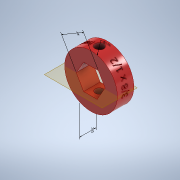
# Autodesk Inventor part: 3_8x1_2-hexBearingSplitA
Saved by Autodesk Inventor 2022.1 (Build 261234000, 234)
## iProperties
Created: 2020-11-08
Part Number: 3_8x1_2-hexBearingSplitA
Material: PC/ABS Plastic
Document SubType Name: Modeling
Designer: robst
Density: 0.357273 g/cm^3
Appearance: Red
Author: robst
Autodesk Inventor part; units mm, degrees
ref_plane "YZ Plane" through (0, 0, 0) normal (1, 0, 0) x (0, 1, 0)
ref_plane "XY Plane" through (0, 0, 0) normal (0, 0, 1) x (1, 0, 0)
sketch "Sketch1" plane through (0, 0, 0) normal (0, 0, 1) x (1, 0, 0)
  line L0 (3.6662, 6.35) -> (7.3323, 0)
  line L1 (7.3323, 0) -> (3.6662, -6.35)
  line L2 (3.6662, -6.35) -> (-3.6662, -6.35)
  line L3 (-3.6662, -6.35) -> (-7.3323, 0)
  line L4 (-7.3323, 0) -> (-3.6662, 6.35)
  line L5 (-3.6662, 6.35) -> (3.6662, 6.35)
  circle A0 centre (0, 0) radius 14.2875
  circle A1 centre (0, 0) radius 7.3323 construction
  dimension "d0" = 12.7
  dimension "d2" = 28.575
  dimension "d3" = 6.9551
  constraints: 12 end point, 3 coincident, 1 centre point, 1 horizontal, 1 horizontal alignment, 15 other
  measures "d0" distance between parallel lines of L2 L5
  measures "d2" diameter of A0
extrude "Extrusion1" add sketch "Sketch1" against normal blind 9.525
thicken "Thicken2" operation add thickness 0.5715 both sides no extend neighbours yes toward (-0.8660254, -0.5, 0) faces at (-4.8882, -4.2333, -3.175) (-6.1103, 2.1167, -3.175) (-1.2221, 6.35, -3.175) (4.8882, 4.2333, -3.175) (7.8832, 4.3299, 0) (1.2221, -6.35, -3.175)
ref_plane "Work Plane1" through (0, 14.2875, 0) normal (0, 1, 0) x (-1, 0, 0)
sketch "Sketch2" plane through (0, 14.2875, 0) normal (0, 1, 0) x (-1, 0, 0)
  line L0 (0, -6.9215) -> (-25.4, -6.9215) construction
  line L1 (14.2875, -0.5715) -> (-14.2875, -0.5715) construction
  spline S0 degree 2 poles (-24.3116, -3.4125) (-24.4274, -3.4125) (-24.6564, -3.4691) (-24.7671, -3.5129) knots 0 0 0 1 2 2 2
  spline S1 degree 2 poles (-24.7671, -3.5129) (-24.87, -3.5566) (-25.0218, -3.6492) (-25.081, -3.6904) knots 0 0 0 1 2 2 2
  line L2 (-25.081, -3.6904) -> (-25.1067, -3.6904)
  line L3 (-25.1067, -3.6904) -> (-25.1067, -3.2401)
  spline S2 degree 2 poles (-25.1067, -3.2401) (-24.9677, -3.1655) (-24.4918, -3.0446) (-24.2782, -3.0446) knots 0 0 0 1 2 2 2
  spline S3 degree 2 poles (-24.2782, -3.0446) (-24.0621, -3.0446) (-23.7405, -3.1321) (-23.6092, -3.2247) knots 0 0 0 1 2 2 2
  spline S4 degree 2 poles (-23.6092, -3.2247) (-23.4703, -3.3251) (-23.3262, -3.6158) (-23.3262, -3.8113) knots 0 0 0 1 2 2 2
  spline S5 degree 2 poles (-23.3262, -3.8113) (-23.3262, -4.0738) (-23.671, -4.47) (-23.9128, -4.5215) knots 0 0 0 1 2 2 2
  line L4 (-23.9128, -4.5215) -> (-23.9128, -4.5523)
  spline S6 degree 2 poles (-23.9128, -4.5523) (-23.8125, -4.5729) (-23.5835, -4.6656) (-23.4857, -4.7582) knots 0 0 0 1 2 2 2
  spline S7 degree 2 poles (-23.4857, -4.7582) (-23.388, -4.8482) (-23.2645, -5.1364) (-23.2645, -5.3448) knots 0 0 0 1 2 2 2
  spline S8 degree 2 poles (-23.2645, -5.3448) (-23.2645, -5.5584) (-23.4111, -5.9211) (-23.5449, -6.0601) knots 0 0 0 1 2 2 2
  spline S9 degree 2 poles (-23.5449, -6.0601) (-23.6839, -6.2042) (-24.0775, -6.3534) (-24.3271, -6.3534) knots 0 0 0 1 2 2 2
  spline S10 degree 2 poles (-24.3271, -6.3534) (-24.5664, -6.3534) (-25.0346, -6.2376) (-25.1942, -6.1579) knots 0 0 0 1 2 2 2
  line L5 (-25.1942, -6.1579) -> (-25.1942, -5.7076)
  line L6 (-25.1942, -5.7076) -> (-25.1633, -5.7076)
  spline S11 degree 2 poles (-25.1633, -5.7076) (-25.0295, -5.8054) (-24.5767, -5.9855) (-24.3528, -5.9855) knots 0 0 0 1 2 2 2
  spline S12 degree 2 poles (-24.3528, -5.9855) (-24.2216, -5.9855) (-23.9592, -5.9031) (-23.8717, -5.8079) knots 0 0 0 1 2 2 2
  spline S13 degree 2 poles (-23.8717, -5.8079) (-23.7868, -5.7127) (-23.6967, -5.4863) (-23.6967, -5.3139) knots 0 0 0 1 2 2 2
  spline S14 degree 2 poles (-23.6967, -5.3139) (-23.6967, -5.1415) (-23.7971, -4.9177) (-23.8871, -4.8534) knots 0 0 0 1 2 2 2
  spline S15 degree 2 poles (-23.8871, -4.8534) (-23.9772, -4.7891) (-24.2216, -4.7402) (-24.3657, -4.7402) knots 0 0 0 1 2 2 2
  line L7 (-24.3657, -4.7402) -> (-24.5458, -4.7402)
  line L8 (-24.5458, -4.7402) -> (-24.5458, -4.3877)
  line L9 (-24.5458, -4.3877) -> (-24.4043, -4.3877)
  spline S16 degree 2 poles (-24.4043, -4.3877) (-24.1187, -4.3877) (-23.7585, -4.1149) (-23.7585, -3.8551) knots 0 0 0 1 2 2 2
  spline S17 degree 2 poles (-23.7585, -3.8551) (-23.7585, -3.7341) (-23.8511, -3.5618) (-23.9257, -3.5103) knots 0 0 0 1 2 2 2
  spline S18 degree 2 poles (-23.9257, -3.5103) (-24.0055, -3.4563) (-24.201, -3.4125) (-24.3116, -3.4125) knots 0 0 0 1 2 2 2
  line L10 (-21.466, -2.97) -> (-22.7087, -6.976)
  line L11 (-22.7087, -6.976) -> (-23.0689, -6.976)
  line L12 (-23.0689, -6.976) -> (-21.8313, -2.97)
  line L13 (-21.8313, -2.97) -> (-21.466, -2.97)
  spline S19 degree 2 poles (-20.1564, -6.3585) (-20.3931, -6.3585) (-20.7816, -6.217) (-20.9179, -6.0858) knots 0 0 0 1 2 2 2
  spline S20 degree 2 poles (-20.9179, -6.0858) (-21.0517, -5.9572) (-21.1907, -5.6072) (-21.1907, -5.4091) knots 0 0 0 1 2 2 2
  spline S21 degree 2 poles (-21.1907, -5.4091) (-21.1907, -5.1518) (-20.9154, -4.7196) (-20.6529, -4.5909) knots 0 0 0 1 2 2 2
  line L14 (-20.6529, -4.5909) -> (-20.6529, -4.5781)
  spline S22 degree 2 poles (-20.6529, -4.5781) (-20.8871, -4.4417) (-21.1135, -4.1175) (-21.1135, -3.8757) knots 0 0 0 1 2 2 2
  spline S23 degree 2 poles (-21.1135, -3.8757) (-21.1135, -3.518) (-20.5732, -3.0395) (-20.1564, -3.0395) knots 0 0 0 1 2 2 2
  spline S24 degree 2 poles (-20.1564, -3.0395) (-19.7241, -3.0395) (-19.2018, -3.4923) (-19.2018, -3.8474) knots 0 0 0 1 2 2 2
  spline S25 degree 2 poles (-19.2018, -3.8474) (-19.2018, -4.0609) (-19.4514, -4.4777) (-19.6855, -4.5961) knots 0 0 0 1 2 2 2
  line L15 (-19.6855, -4.5961) -> (-19.6855, -4.6089)
  spline S26 degree 2 poles (-19.6855, -4.6089) (-19.4076, -4.7376) (-19.122, -5.1081) (-19.122, -5.4014) knots 0 0 0 1 2 2 2
  spline S27 degree 2 poles (-19.122, -5.4014) (-19.122, -5.8079) (-19.7138, -6.3585) (-20.1564, -6.3585) knots 0 0 0 1 2 2 2
  spline S28 degree 2 poles (-19.5594, -5.4426) (-19.5594, -5.247) (-19.7138, -5.0155) (-19.9325, -4.8971) knots 0 0 0 1 2 2 2
  spline S29 degree 2 poles (-19.9325, -4.8971) (-20.0046, -4.8559) (-20.2464, -4.7608) (-20.3982, -4.699) knots 0 0 0 1 2 2 2
  spline S30 degree 2 poles (-20.3982, -4.699) (-20.5732, -4.8148) (-20.761, -5.1596) (-20.761, -5.3783) knots 0 0 0 1 2 2 2
  spline S31 degree 2 poles (-20.761, -5.3783) (-20.761, -5.6664) (-20.4137, -6.0421) (-20.1512, -6.0421) knots 0 0 0 1 2 2 2
  spline S32 degree 2 poles (-20.1512, -6.0421) (-19.8836, -6.0421) (-19.5594, -5.7205) (-19.5594, -5.4426) knots 0 0 0 1 2 2 2
  spline S33 degree 2 poles (-19.6186, -3.8525) (-19.6186, -3.639) (-19.9042, -3.3534) (-20.1589, -3.3534) knots 0 0 0 1 2 2 2
  spline S34 degree 2 poles (-20.1589, -3.3534) (-20.3905, -3.3534) (-20.6864, -3.6081) (-20.6864, -3.8268) knots 0 0 0 1 2 2 2
  spline S35 degree 2 poles (-20.6864, -3.8268) (-20.6864, -3.9837) (-20.5346, -4.2024) (-20.3828, -4.2899) knots 0 0 0 1 2 2 2
  spline S36 degree 2 poles (-20.3828, -4.2899) (-20.3185, -4.3259) (-20.0457, -4.452) (-19.9351, -4.488) knots 0 0 0 1 2 2 2
  spline S37 degree 2 poles (-19.9351, -4.488) (-19.7498, -4.3465) (-19.6186, -4.0455) (-19.6186, -3.8525) knots 0 0 0 1 2 2 2
  line L16 (-15.4608, -6.2865) -> (-15.9522, -6.2865)
  line L17 (-15.9522, -6.2865) -> (-16.5311, -5.3911)
  line L18 (-16.5311, -5.3911) -> (-17.1254, -6.2865)
  line L19 (-17.1254, -6.2865) -> (-17.5809, -6.2865)
  line L20 (-17.5809, -6.2865) -> (-16.7549, -5.1055)
  line L21 (-16.7549, -5.1055) -> (-17.5731, -3.904)
  line L22 (-17.5731, -3.904) -> (-17.0817, -3.904)
  line L23 (-17.0817, -3.904) -> (-16.5054, -4.7916)
  line L24 (-16.5054, -4.7916) -> (-15.9162, -3.904)
  line L25 (-15.9162, -3.904) -> (-15.4608, -3.904)
  line L26 (-15.4608, -3.904) -> (-16.2815, -5.0798)
  line L27 (-16.2815, -5.0798) -> (-15.4608, -6.2865)
  line L28 (-12.0465, -6.2865) -> (-13.5954, -6.2865)
  line L29 (-13.5954, -6.2865) -> (-13.5954, -5.9623)
  line L30 (-13.5954, -5.9623) -> (-13.019, -5.9623)
  line L31 (-13.019, -5.9623) -> (-13.019, -3.8345)
  line L32 (-13.019, -3.8345) -> (-13.5954, -3.8345)
  line L33 (-13.5954, -3.8345) -> (-13.5954, -3.5438)
  spline S38 degree 2 poles (-13.5954, -3.5438) (-13.2686, -3.5438) (-12.9599, -3.3585) (-12.9393, -3.1012) knots 0 0 0 1 2 2 2
  line L34 (-12.9393, -3.1012) -> (-12.6099, -3.1012)
  line L35 (-12.6099, -3.1012) -> (-12.6099, -5.9623)
  line L36 (-12.6099, -5.9623) -> (-12.0465, -5.9623)
  line L37 (-12.0465, -5.9623) -> (-12.0465, -6.2865)
  line L38 (-10.1425, -2.97) -> (-11.3852, -6.976)
  line L39 (-11.3852, -6.976) -> (-11.7454, -6.976)
  line L40 (-11.7454, -6.976) -> (-10.5079, -2.97)
  line L41 (-10.5079, -2.97) -> (-10.1425, -2.97)
  line L42 (-7.8346, -6.2865) -> (-9.7926, -6.2865)
  line L43 (-9.7926, -6.2865) -> (-9.7926, -5.8362)
  spline S39 degree 2 poles (-9.7926, -5.8362) (-9.5816, -5.6381) (-9.206, -5.2702) (-9.0259, -5.0721) knots 0 0 0 1 2 2 2
  spline S40 degree 2 poles (-9.0259, -5.0721) (-8.6631, -4.6733) (-8.3981, -4.1947) (-8.3981, -3.94) knots 0 0 0 1 2 2 2
  spline S41 degree 2 poles (-8.3981, -3.94) (-8.3981, -3.8062) (-8.4804, -3.6055) (-8.555, -3.5412) knots 0 0 0 1 2 2 2
  spline S42 degree 2 poles (-8.555, -3.5412) (-8.6296, -3.4769) (-8.8252, -3.4125) (-8.9435, -3.4125) knots 0 0 0 1 2 2 2
  spline S43 degree 2 poles (-8.9435, -3.4125) (-9.0567, -3.4125) (-9.2883, -3.4691) (-9.3938, -3.5129) knots 0 0 0 1 2 2 2
  spline S44 degree 2 poles (-9.3938, -3.5129) (-9.4838, -3.5489) (-9.6511, -3.6518) (-9.7025, -3.6878) knots 0 0 0 1 2 2 2
  line L44 (-9.7025, -3.6878) -> (-9.7257, -3.6878)
  line L45 (-9.7257, -3.6878) -> (-9.7257, -3.235)
  spline S45 degree 2 poles (-9.7257, -3.235) (-9.5945, -3.1707) (-9.1236, -3.0446) (-8.9126, -3.0446) knots 0 0 0 1 2 2 2
  spline S46 degree 2 poles (-8.9126, -3.0446) (-8.4675, -3.0446) (-7.9658, -3.5155) (-7.9658, -3.9168) knots 0 0 0 1 2 2 2
  spline S47 degree 2 poles (-7.9658, -3.9168) (-7.9658, -4.1047) (-8.0533, -4.4186) (-8.1305, -4.5523) knots 0 0 0 1 2 2 2
  spline S48 degree 2 poles (-8.1305, -4.5523) (-8.2077, -4.6913) (-8.4315, -4.964) (-8.555, -5.0952) knots 0 0 0 1 2 2 2
  spline S49 degree 2 poles (-8.555, -5.0952) (-8.7557, -5.3139) (-9.2471, -5.7822) (-9.3938, -5.9186) knots 0 0 0 1 2 2 2
  line L46 (-9.3938, -5.9186) -> (-7.8346, -5.9186)
  line L47 (-7.8346, -5.9186) -> (-7.8346, -6.2865)
  line L48 (5.4289, -6.2865) -> (5.0275, -6.2865)
  line L49 (5.0275, -6.2865) -> (5.0275, -4.928)
  spline S50 degree 2 poles (5.0275, -4.928) (5.0275, -4.7633) (4.9966, -4.4803) (4.9503, -4.3954) knots 0 0 0 1 2 2 2
  spline S51 degree 2 poles (4.9503, -4.3954) (4.9014, -4.3053) (4.7265, -4.2179) (4.5772, -4.2179) knots 0 0 0 1 2 2 2
  spline S52 degree 2 poles (4.5772, -4.2179) (4.428, -4.2179) (4.1115, -4.3774) (3.9597, -4.506) knots 0 0 0 1 2 2 2
  line L50 (3.9597, -4.506) -> (3.9597, -6.2865)
  line L51 (3.9597, -6.2865) -> (3.5584, -6.2865)
  line L52 (3.5584, -6.2865) -> (3.5584, -2.97)
  line L53 (3.5584, -2.97) -> (3.9597, -2.97)
  line L54 (3.9597, -2.97) -> (3.9597, -4.169)
  spline S53 degree 2 poles (3.9597, -4.169) (4.1398, -4.0069) (4.4872, -3.8371) (4.6827, -3.8371) knots 0 0 0 1 2 2 2
  spline S54 degree 2 poles (4.6827, -3.8371) (5.0327, -3.8371) (5.4289, -4.3002) (5.4289, -4.7402) knots 0 0 0 1 2 2 2
  line L55 (5.4289, -4.7402) -> (5.4289, -6.2865)
  spline S55 degree 2 poles (7.0267, -6.3405) (6.4555, -6.3405) (5.8277, -5.6999) (5.8277, -5.1081) knots 0 0 0 1 2 2 2
  spline S56 degree 2 poles (5.8277, -5.1081) (5.8277, -4.5266) (6.4375, -3.8371) (6.9289, -3.8371) knots 0 0 0 1 2 2 2
  spline S57 degree 2 poles (6.9289, -3.8371) (7.1502, -3.8371) (7.4924, -3.9657) (7.6185, -4.1021) knots 0 0 0 1 2 2 2
  spline S58 degree 2 poles (7.6185, -4.1021) (7.7471, -4.2384) (7.8835, -4.6321) (7.8835, -4.9177) knots 0 0 0 1 2 2 2
  line L56 (7.8835, -4.9177) -> (7.8835, -5.1364)
  line L57 (7.8835, -5.1364) -> (6.2342, -5.1364)
  spline S59 degree 2 poles (6.2342, -5.1364) (6.2342, -5.5506) (6.651, -5.9906) (7.0215, -5.9906) knots 0 0 0 1 2 2 2
  spline S60 degree 2 poles (7.0215, -5.9906) (7.1528, -5.9906) (7.4075, -5.9314) (7.5104, -5.8851) knots 0 0 0 1 2 2 2
  spline S61 degree 2 poles (7.5104, -5.8851) (7.6185, -5.8337) (7.7677, -5.7436) (7.8166, -5.7024) knots 0 0 0 1 2 2 2
  line L58 (7.8166, -5.7024) -> (7.8397, -5.7024)
  line L59 (7.8397, -5.7024) -> (7.8397, -6.1398)
  spline S62 degree 2 poles (7.8397, -6.1398) (7.7703, -6.1681) (7.5593, -6.2505) (7.4769, -6.2736) knots 0 0 0 1 2 2 2
  spline S63 degree 2 poles (7.4769, -6.2736) (7.3612, -6.3071) (7.1708, -6.3405) (7.0267, -6.3405) knots 0 0 0 1 2 2 2
  spline S64 degree 2 poles (7.4924, -4.8302) (7.4872, -4.6681) (7.4203, -4.4314) (7.356, -4.3517) knots 0 0 0 1 2 2 2
  spline S65 degree 2 poles (7.356, -4.3517) (7.2865, -4.2616) (7.0678, -4.1664) (6.9058, -4.1664) knots 0 0 0 1 2 2 2
  spline S66 degree 2 poles (6.9058, -4.1664) (6.7462, -4.1664) (6.5224, -4.2616) (6.4298, -4.3542) knots 0 0 0 1 2 2 2
  spline S67 degree 2 poles (6.4298, -4.3542) (6.3397, -4.4494) (6.2471, -4.6784) (6.2342, -4.8302) knots 0 0 0 1 2 2 2
  line L60 (6.2342, -4.8302) -> (7.4924, -4.8302)
  line L61 (10.1399, -6.2865) -> (9.6485, -6.2865)
  line L62 (9.6485, -6.2865) -> (9.0696, -5.3911)
  line L63 (9.0696, -5.3911) -> (8.4752, -6.2865)
  line L64 (8.4752, -6.2865) -> (8.0198, -6.2865)
  line L65 (8.0198, -6.2865) -> (8.8457, -5.1055)
  line L66 (8.8457, -5.1055) -> (8.0276, -3.904)
  line L67 (8.0276, -3.904) -> (8.519, -3.904)
  line L68 (8.519, -3.904) -> (9.0953, -4.7916)
  line L69 (9.0953, -4.7916) -> (9.6845, -3.904)
  line L70 (9.6845, -3.904) -> (10.1399, -3.904)
  line L71 (10.1399, -3.904) -> (9.3192, -5.0798)
  line L72 (9.3192, -5.0798) -> (10.1399, -6.2865)
  spline S68 degree 2 poles (13.8115, -5.0566) (13.8115, -5.6407) (13.2455, -6.3534) (12.8184, -6.3534) knots 0 0 0 1 2 2 2
  spline S69 degree 2 poles (12.8184, -6.3534) (12.6254, -6.3534) (12.3501, -6.2582) (12.2163, -6.1759) knots 0 0 0 1 2 2 2
  line L73 (12.2163, -6.1759) -> (12.1906, -6.2865)
  line L74 (12.1906, -6.2865) -> (11.8149, -6.2865)
  line L75 (11.8149, -6.2865) -> (11.8149, -2.97)
  line L76 (11.8149, -2.97) -> (12.2163, -2.97)
  line L77 (12.2163, -2.97) -> (12.2163, -4.1535)
  spline S70 degree 2 poles (12.2163, -4.1535) (12.3681, -4.0172) (12.7206, -3.8371) (12.9444, -3.8371) knots 0 0 0 1 2 2 2
  spline S71 degree 2 poles (12.9444, -3.8371) (13.3484, -3.8371) (13.8115, -4.4829) (13.8115, -5.0566) knots 0 0 0 1 2 2 2
  spline S72 degree 2 poles (13.3973, -5.0875) (13.3973, -4.6604) (13.1374, -4.2179) (12.8492, -4.2179) knots 0 0 0 1 2 2 2
  spline S73 degree 2 poles (12.8492, -4.2179) (12.6871, -4.2179) (12.3527, -4.3722) (12.2163, -4.4906) knots 0 0 0 1 2 2 2
  line L78 (12.2163, -4.4906) -> (12.2163, -5.8568)
  spline S74 degree 2 poles (12.2163, -5.8568) (12.3681, -5.9314) (12.6022, -5.9932) (12.7412, -5.9932) knots 0 0 0 1 2 2 2
  spline S75 degree 2 poles (12.7412, -5.9932) (13.0473, -5.9932) (13.3973, -5.5584) (13.3973, -5.0875) knots 0 0 0 1 2 2 2
  line L79 (16.0808, -6.2865) -> (15.6795, -6.2865)
  line L80 (15.6795, -6.2865) -> (15.6795, -6.0241)
  spline S76 degree 2 poles (15.6795, -6.0241) (15.4942, -6.1862) (15.1623, -6.3534) (14.9565, -6.3534) knots 0 0 0 1 2 2 2
  spline S77 degree 2 poles (14.9565, -6.3534) (14.8021, -6.3534) (14.5268, -6.2505) (14.4264, -6.1398) knots 0 0 0 1 2 2 2
  spline S78 degree 2 poles (14.4264, -6.1398) (14.3235, -6.0292) (14.2103, -5.6922) (14.2103, -5.4503) knots 0 0 0 1 2 2 2
  line L81 (14.2103, -5.4503) -> (14.2103, -3.904)
  line L82 (14.2103, -3.904) -> (14.6117, -3.904)
  line L83 (14.6117, -3.904) -> (14.6117, -5.2625)
  spline S79 degree 2 poles (14.6117, -5.2625) (14.6117, -5.4529) (14.64, -5.7024) (14.6889, -5.7951) knots 0 0 0 1 2 2 2
  spline S80 degree 2 poles (14.6889, -5.7951) (14.7378, -5.8877) (14.905, -5.9726) (15.062, -5.9726) knots 0 0 0 1 2 2 2
  spline S81 degree 2 poles (15.062, -5.9726) (15.2086, -5.9726) (15.5405, -5.8054) (15.6795, -5.6844) knots 0 0 0 1 2 2 2
  line L84 (15.6795, -5.6844) -> (15.6795, -3.904)
  line L85 (15.6795, -3.904) -> (16.0808, -3.904)
  line L86 (16.0808, -3.904) -> (16.0808, -6.2865)
  spline S82 degree 2 poles (17.3055, -6.3431) (17.0663, -6.3431) (16.652, -6.2145) (16.5157, -6.1424) knots 0 0 0 1 2 2 2
  line L87 (16.5157, -6.1424) -> (16.5157, -5.6922)
  line L88 (16.5157, -5.6922) -> (16.5362, -5.6922)
  spline S83 degree 2 poles (16.5362, -5.6922) (16.5877, -5.7333) (16.7266, -5.8311) (16.8424, -5.8851) knots 0 0 0 1 2 2 2
  spline S84 degree 2 poles (16.8424, -5.8851) (16.9428, -5.934) (17.1898, -6.0061) (17.321, -6.0061) knots 0 0 0 1 2 2 2
  spline S85 degree 2 poles (17.321, -6.0061) (17.4162, -6.0061) (17.6349, -5.9623) (17.6863, -5.9263) knots 0 0 0 1 2 2 2
  spline S86 degree 2 poles (17.6863, -5.9263) (17.761, -5.8774) (17.8279, -5.7668) (17.8279, -5.6536) knots 0 0 0 1 2 2 2
  spline S87 degree 2 poles (17.8279, -5.6536) (17.8279, -5.512) (17.6735, -5.3654) (17.4754, -5.3165) knots 0 0 0 1 2 2 2
  spline S88 degree 2 poles (17.4754, -5.3165) (17.3982, -5.2985) (17.1512, -5.247) (17.0457, -5.2187) knots 0 0 0 1 2 2 2
  spline S89 degree 2 poles (17.0457, -5.2187) (16.773, -5.139) (16.526, -4.8096) (16.526, -4.5755) knots 0 0 0 1 2 2 2
  spline S90 degree 2 poles (16.526, -4.5755) (16.526, -4.2513) (17.0122, -3.8474) (17.4136, -3.8474) knots 0 0 0 1 2 2 2
  spline S91 degree 2 poles (17.4136, -3.8474) (17.6117, -3.8474) (18.0131, -3.9451) (18.1495, -4.0197) knots 0 0 0 1 2 2 2
  line L89 (18.1495, -4.0197) -> (18.1495, -4.4494)
  line L90 (18.1495, -4.4494) -> (18.1289, -4.4494)
  spline S92 degree 2 poles (18.1289, -4.4494) (17.9745, -4.3259) (17.5989, -4.1844) (17.4059, -4.1844) knots 0 0 0 1 2 2 2
  spline S93 degree 2 poles (17.4059, -4.1844) (17.2078, -4.1844) (16.935, -4.3517) (16.935, -4.5189) knots 0 0 0 1 2 2 2
  spline S94 degree 2 poles (16.935, -4.5189) (16.935, -4.6707) (17.0971, -4.8174) (17.2772, -4.8637) knots 0 0 0 1 2 2 2
  spline S95 degree 2 poles (17.2772, -4.8637) (17.3647, -4.8868) (17.586, -4.9331) (17.7069, -4.9614) knots 0 0 0 1 2 2 2
  spline S96 degree 2 poles (17.7069, -4.9614) (17.9694, -5.0283) (18.237, -5.3345) (18.237, -5.5995) knots 0 0 0 1 2 2 2
  spline S97 degree 2 poles (18.237, -5.5995) (18.237, -5.7539) (18.116, -6.0266) (17.9977, -6.127) knots 0 0 0 1 2 2 2
  spline S98 degree 2 poles (17.9977, -6.127) (17.8716, -6.2325) (17.55, -6.3431) (17.3055, -6.3431) knots 0 0 0 1 2 2 2
  line L91 (20.4805, -6.2865) -> (20.0792, -6.2865)
  line L92 (20.0792, -6.2865) -> (20.0792, -4.928)
  spline S99 degree 2 poles (20.0792, -4.928) (20.0792, -4.7633) (20.0483, -4.4803) (20.002, -4.3954) knots 0 0 0 1 2 2 2
  spline S100 degree 2 poles (20.002, -4.3954) (19.9531, -4.3053) (19.7781, -4.2179) (19.6289, -4.2179) knots 0 0 0 1 2 2 2
  spline S101 degree 2 poles (19.6289, -4.2179) (19.4797, -4.2179) (19.1632, -4.3774) (19.0114, -4.506) knots 0 0 0 1 2 2 2
  line L93 (19.0114, -4.506) -> (19.0114, -6.2865)
  line L94 (19.0114, -6.2865) -> (18.61, -6.2865)
  line L95 (18.61, -6.2865) -> (18.61, -2.97)
  line L96 (18.61, -2.97) -> (19.0114, -2.97)
  line L97 (19.0114, -2.97) -> (19.0114, -4.169)
  spline S102 degree 2 poles (19.0114, -4.169) (19.1915, -4.0069) (19.5389, -3.8371) (19.7344, -3.8371) knots 0 0 0 1 2 2 2
  spline S103 degree 2 poles (19.7344, -3.8371) (20.0843, -3.8371) (20.4805, -4.3002) (20.4805, -4.7402) knots 0 0 0 1 2 2 2
  line L98 (20.4805, -4.7402) -> (20.4805, -6.2865)
  line L99 (21.4531, -6.2865) -> (21.0517, -6.2865)
  line L100 (21.0517, -6.2865) -> (21.0517, -3.904)
  line L101 (21.0517, -3.904) -> (21.4531, -3.904)
  line L102 (21.4531, -3.904) -> (21.4531, -6.2865)
  line L103 (21.4814, -3.5077) -> (21.026, -3.5077)
  line L104 (21.026, -3.5077) -> (21.026, -3.0909)
  line L105 (21.026, -3.0909) -> (21.4814, -3.0909)
  line L106 (21.4814, -3.0909) -> (21.4814, -3.5077)
  line L107 (23.9128, -6.2865) -> (23.5115, -6.2865)
  line L108 (23.5115, -6.2865) -> (23.5115, -4.928)
  spline S104 degree 2 poles (23.5115, -4.928) (23.5115, -4.7633) (23.4806, -4.4803) (23.4343, -4.3954) knots 0 0 0 1 2 2 2
  spline S105 degree 2 poles (23.4343, -4.3954) (23.3854, -4.3053) (23.2104, -4.2179) (23.0612, -4.2179) knots 0 0 0 1 2 2 2
  spline S106 degree 2 poles (23.0612, -4.2179) (22.912, -4.2179) (22.5955, -4.3774) (22.4437, -4.506) knots 0 0 0 1 2 2 2
  line L109 (22.4437, -4.506) -> (22.4437, -6.2865)
  line L110 (22.4437, -6.2865) -> (22.0423, -6.2865)
  line L111 (22.0423, -6.2865) -> (22.0423, -3.904)
  line L112 (22.0423, -3.904) -> (22.4437, -3.904)
  line L113 (22.4437, -3.904) -> (22.4437, -4.169)
  spline S107 degree 2 poles (22.4437, -4.169) (22.6238, -4.0069) (22.9711, -3.8371) (23.1667, -3.8371) knots 0 0 0 1 2 2 2
  spline S108 degree 2 poles (23.1667, -3.8371) (23.5166, -3.8371) (23.9128, -4.3002) (23.9128, -4.7402) knots 0 0 0 1 2 2 2
  line L114 (23.9128, -4.7402) -> (23.9128, -6.2865)
  spline S109 degree 2 poles (24.5612, -6.6673) (24.6024, -6.6853) (24.7593, -6.7419) (24.8597, -6.7651) knots 0 0 0 1 2 2 2
  spline S110 degree 2 poles (24.8597, -6.7651) (24.9703, -6.7934) (25.1581, -6.8268) (25.2688, -6.8268) knots 0 0 0 1 2 2 2
  spline S111 degree 2 poles (25.2688, -6.8268) (25.454, -6.8268) (25.7113, -6.729) (25.7834, -6.6416) knots 0 0 0 1 2 2 2
  spline S112 degree 2 poles (25.7834, -6.6416) (25.8528, -6.5541) (25.9069, -6.3251) (25.9069, -6.1784) knots 0 0 0 1 2 2 2
  line L115 (25.9069, -6.1784) -> (25.9069, -5.97)
  spline S113 degree 2 poles (25.9069, -5.97) (25.7448, -6.1115) (25.4334, -6.2453) (25.1993, -6.2453) knots 0 0 0 1 2 2 2
  spline S114 degree 2 poles (25.1993, -6.2453) (24.7928, -6.2453) (24.3116, -5.6407) (24.3116, -5.0721) knots 0 0 0 1 2 2 2
  spline S115 degree 2 poles (24.3116, -5.0721) (24.3116, -4.7762) (24.4789, -4.3182) (24.6178, -4.1561) knots 0 0 0 1 2 2 2
  spline S116 degree 2 poles (24.6178, -4.1561) (24.7516, -4.0043) (25.1195, -3.8371) (25.3151, -3.8371) knots 0 0 0 1 2 2 2
  spline S117 degree 2 poles (25.3151, -3.8371) (25.5003, -3.8371) (25.7705, -3.9245) (25.9069, -4.0043) knots 0 0 0 1 2 2 2
  line L116 (25.9069, -4.0043) -> (25.93, -3.904)
  line L117 (25.93, -3.904) -> (26.3082, -3.904)
  line L118 (26.3082, -3.904) -> (26.3082, -6.0138)
  spline S118 degree 2 poles (26.3082, -6.0138) (26.3082, -6.621) (25.7808, -7.187) (25.2379, -7.187) knots 0 0 0 1 2 2 2
  spline S119 degree 2 poles (25.2379, -7.187) (25.0629, -7.187) (24.6976, -7.1304) (24.5406, -7.0841) knots 0 0 0 1 2 2 2
  line L119 (24.5406, -7.0841) -> (24.5406, -6.6673)
  line L120 (24.5406, -6.6673) -> (24.5612, -6.6673)
  line L121 (25.9069, -5.6407) -> (25.9069, -4.3311)
  spline S120 degree 2 poles (25.9069, -4.3311) (25.7576, -4.259) (25.5055, -4.1973) (25.3794, -4.1973) knots 0 0 0 1 2 2 2
  spline S121 degree 2 poles (25.3794, -4.1973) (25.0758, -4.1973) (24.7259, -4.645) (24.7259, -5.0644) knots 0 0 0 1 2 2 2
  spline S122 degree 2 poles (24.7259, -5.0644) (24.7259, -5.4606) (24.9909, -5.8748) (25.2894, -5.8748) knots 0 0 0 1 2 2 2
  spline S123 degree 2 poles (25.2894, -5.8748) (25.4463, -5.8748) (25.7756, -5.7513) (25.9069, -5.6407) knots 0 0 0 1 2 2 2
  spline S124 degree 2 poles (30.25, -5.0309) (30.25, -5.6278) (29.6814, -6.3328) (29.2465, -6.3328) knots 0 0 0 1 2 2 2
  spline S125 degree 2 poles (29.2465, -6.3328) (29.069, -6.3328) (28.7963, -6.2505) (28.6548, -6.1656) knots 0 0 0 1 2 2 2
  line L122 (28.6548, -6.1656) -> (28.6548, -7.1639)
  line L123 (28.6548, -7.1639) -> (28.2534, -7.1639)
  line L124 (28.2534, -7.1639) -> (28.2534, -3.904)
  line L125 (28.2534, -3.904) -> (28.6548, -3.904)
  line L126 (28.6548, -3.904) -> (28.6548, -4.1535)
  spline S126 degree 2 poles (28.6548, -4.1535) (28.804, -4.0172) (29.1693, -3.8371) (29.3829, -3.8371) knots 0 0 0 1 2 2 2
  spline S127 degree 2 poles (29.3829, -3.8371) (29.792, -3.8371) (30.25, -4.4854) (30.25, -5.0309) knots 0 0 0 1 2 2 2
  spline S128 degree 2 poles (29.8357, -5.0772) (29.8357, -4.6681) (29.5759, -4.2179) (29.2851, -4.2179) knots 0 0 0 1 2 2 2
  spline S129 degree 2 poles (29.2851, -4.2179) (29.1153, -4.2179) (28.7963, -4.3697) (28.6548, -4.488) knots 0 0 0 1 2 2 2
  line L127 (28.6548, -4.488) -> (28.6548, -5.8414)
  spline S130 degree 2 poles (28.6548, -5.8414) (28.8117, -5.916) (29.0356, -5.9726) (29.1796, -5.9726) knots 0 0 0 1 2 2 2
  spline S131 degree 2 poles (29.1796, -5.9726) (29.491, -5.9726) (29.8357, -5.5146) (29.8357, -5.0772) knots 0 0 0 1 2 2 2
  line L128 (32.5373, -3.904) -> (31.6394, -6.2865)
  line L129 (31.6394, -6.2865) -> (31.2792, -6.2865)
  line L130 (31.2792, -6.2865) -> (30.3889, -3.904)
  line L131 (30.3889, -3.904) -> (30.8237, -3.904)
  line L132 (30.8237, -3.904) -> (31.4747, -5.7385)
  line L133 (31.4747, -5.7385) -> (32.1205, -3.904)
  line L134 (32.1205, -3.904) -> (32.5373, -3.904)
  spline S132 degree 2 poles (34.7578, -4.699) (34.7578, -5.5532) (34.2612, -6.3534) (33.744, -6.3534) knots 0 0 0 1 2 2 2
  spline S133 degree 2 poles (33.744, -6.3534) (33.2191, -6.3534) (32.7277, -5.5378) (32.7277, -4.7016) knots 0 0 0 1 2 2 2
  spline S134 degree 2 poles (32.7277, -4.7016) (32.7277, -3.8422) (33.2243, -3.0472) (33.744, -3.0472) knots 0 0 0 1 2 2 2
  spline S135 degree 2 poles (33.744, -3.0472) (34.2663, -3.0472) (34.7578, -3.8705) (34.7578, -4.699) knots 0 0 0 1 2 2 2
  spline S136 degree 2 poles (34.2123, -5.6664) (34.274, -5.5095) (34.3255, -5.0258) (34.3255, -4.699) knots 0 0 0 1 2 2 2
  spline S137 degree 2 poles (34.3255, -4.699) (34.3255, -4.3722) (34.274, -3.8911) (34.2097, -3.729) knots 0 0 0 1 2 2 2
  spline S138 degree 2 poles (34.2097, -3.729) (34.1454, -3.5669) (33.9216, -3.3997) (33.744, -3.3997) knots 0 0 0 1 2 2 2
  spline S139 degree 2 poles (33.744, -3.3997) (33.5665, -3.3997) (33.3375, -3.5669) (33.2706, -3.7341) knots 0 0 0 1 2 2 2
  spline S140 degree 2 poles (33.2706, -3.7341) (33.2063, -3.8962) (33.16, -4.3902) (33.16, -4.7016) knots 0 0 0 1 2 2 2
  spline S141 degree 2 poles (33.16, -4.7016) (33.16, -5.0361) (33.2011, -5.4837) (33.268, -5.6587) knots 0 0 0 1 2 2 2
  spline S142 degree 2 poles (33.268, -5.6587) (33.3298, -5.8234) (33.5588, -6.0009) (33.744, -6.0009) knots 0 0 0 1 2 2 2
  spline S143 degree 2 poles (33.744, -6.0009) (33.919, -6.0009) (34.148, -5.8337) (34.2123, -5.6664) knots 0 0 0 1 2 2 2
  spline S144 degree 2 poles (36.0211, -3.4125) (35.9053, -3.4125) (35.6763, -3.4691) (35.5657, -3.5129) knots 0 0 0 1 2 2 2
  spline S145 degree 2 poles (35.5657, -3.5129) (35.4627, -3.5566) (35.3109, -3.6492) (35.2518, -3.6904) knots 0 0 0 1 2 2 2
  line L135 (35.2518, -3.6904) -> (35.226, -3.6904)
  line L136 (35.226, -3.6904) -> (35.226, -3.2401)
  spline S146 degree 2 poles (35.226, -3.2401) (35.365, -3.1655) (35.841, -3.0446) (36.0545, -3.0446) knots 0 0 0 1 2 2 2
  spline S147 degree 2 poles (36.0545, -3.0446) (36.2706, -3.0446) (36.5923, -3.1321) (36.7235, -3.2247) knots 0 0 0 1 2 2 2
  spline S148 degree 2 poles (36.7235, -3.2247) (36.8624, -3.3251) (37.0065, -3.6158) (37.0065, -3.8113) knots 0 0 0 1 2 2 2
  spline S149 degree 2 poles (37.0065, -3.8113) (37.0065, -4.0738) (36.6617, -4.47) (36.4199, -4.5215) knots 0 0 0 1 2 2 2
  line L137 (36.4199, -4.5215) -> (36.4199, -4.5523)
  spline S150 degree 2 poles (36.4199, -4.5523) (36.5202, -4.5729) (36.7492, -4.6656) (36.847, -4.7582) knots 0 0 0 1 2 2 2
  spline S151 degree 2 poles (36.847, -4.7582) (36.9448, -4.8482) (37.0683, -5.1364) (37.0683, -5.3448) knots 0 0 0 1 2 2 2
  spline S152 degree 2 poles (37.0683, -5.3448) (37.0683, -5.5584) (36.9216, -5.9211) (36.7878, -6.0601) knots 0 0 0 1 2 2 2
  spline S153 degree 2 poles (36.7878, -6.0601) (36.6489, -6.2042) (36.2552, -6.3534) (36.0056, -6.3534) knots 0 0 0 1 2 2 2
  spline S154 degree 2 poles (36.0056, -6.3534) (35.7663, -6.3534) (35.2981, -6.2376) (35.1386, -6.1579) knots 0 0 0 1 2 2 2
  line L138 (35.1386, -6.1579) -> (35.1386, -5.7076)
  line L139 (35.1386, -5.7076) -> (35.1694, -5.7076)
  spline S155 degree 2 poles (35.1694, -5.7076) (35.3032, -5.8054) (35.7561, -5.9855) (35.9799, -5.9855) knots 0 0 0 1 2 2 2
  spline S156 degree 2 poles (35.9799, -5.9855) (36.1111, -5.9855) (36.3736, -5.9031) (36.461, -5.8079) knots 0 0 0 1 2 2 2
  spline S157 degree 2 poles (36.461, -5.8079) (36.5459, -5.7127) (36.636, -5.4863) (36.636, -5.3139) knots 0 0 0 1 2 2 2
  spline S158 degree 2 poles (36.636, -5.3139) (36.636, -5.1415) (36.5357, -4.9177) (36.4456, -4.8534) knots 0 0 0 1 2 2 2
  spline S159 degree 2 poles (36.4456, -4.8534) (36.3555, -4.7891) (36.1111, -4.7402) (35.967, -4.7402) knots 0 0 0 1 2 2 2
  line L140 (35.967, -4.7402) -> (35.7869, -4.7402)
  line L141 (35.7869, -4.7402) -> (35.7869, -4.3877)
  line L142 (35.7869, -4.3877) -> (35.9284, -4.3877)
  spline S160 degree 2 poles (35.9284, -4.3877) (36.214, -4.3877) (36.5742, -4.1149) (36.5742, -3.8551) knots 0 0 0 1 2 2 2
  spline S161 degree 2 poles (36.5742, -3.8551) (36.5742, -3.7341) (36.4816, -3.5618) (36.407, -3.5103) knots 0 0 0 1 2 2 2
  spline S162 degree 2 poles (36.407, -3.5103) (36.3272, -3.4563) (36.1317, -3.4125) (36.0211, -3.4125) knots 0 0 0 1 2 2 2
  point P0 (0, 0)
  dimension "d17" = 25.4
  dimension "d18" = 6.35
  constraints: 2 end point, 2 horizontal
  measures "d17" distance of L0.start L0.end
  measures "d18" distance between parallel lines of L0 L1
emboss "Emboss1" sketch "Sketch2" operation cut depth 2.54 direction (0, -1, 0) wrap yes faces at (14.2412, -1.1497, -6.5405)
sketch "Sketch3" plane through (0, 14.2875, 0) normal (0, 1, 0) x (-1, 0, 0)
  line L0 (-3.9961, -9.525) -> (3.9961, -9.525) construction
  line L1 (0, -9.525) -> (0, -0.5715) construction
  line L2 (3.9961, -0.5715) -> (-3.9961, -0.5715) construction
  line L3 (14.2875, -0.5715) -> (-14.2875, -0.5715) projected
  point P0 (0, 0)
  point P1 (0, -5.0482)
  dimension "d28" = 4.4768
  dimension "d29" = 4.4768
  constraints: 3 midpoint, 2 end point
  measures "d28" distance from line of L3 point (0, -5.048)
  measures "d29" distance from line of point (0, -5.048) L0
hole "Hole1" at (0, 14.2875, -5.0482) direction (0, -1, 0) diameter 4.318 end through all clearance for "Hex Machine Screw" size "#6" standard "Ansi Unified Screw Threads"
sketch "Sketch4" plane through (0, 14.2875, 0) normal (0, 1, 0) x (-1, 0, 0)
  circle A0 centre (0, -5.0482) radius 2.159 projected
  circle A1 centre (0, -5.0482) radius 2.4257
  point P0 (0, 0)
  point P1 (0, -7.1755)
  point P2 (0, -2.8575)
  point P3 (-1.8469, -6.1346)
  point P4 (-1.9236, -4.0361)
  point P5 (-2.0073, -5.8114)
  point P6 (-2.1583, -5.0729)
  point P7 (-1.8311, -3.8726)
  point P8 (-1.971, -4.1353)
  point P9 (-1.7904, -6.223)
  point P10 (0.4573, -2.9065)
  point P11 (-1.6967, -3.6814)
  point P12 (1.6173, -6.4468)
  dimension "d30" = 4.8514
  constraints: 1 centre point, 1 coincident, 5 other
  measures "d30" diameter of A1
extrude "Extrusion2" cut sketch "Sketch4" against normal blind 5.5524 contours A0 | A1
equation "\"d0\" = hexSize"
equation "\"d2\" = externalDiameter"
equation "\"d4\" = thickness"
equation "\"d8\" = printSpacing"
equation "\"d9\" = printSpacing"
equation "\"hexSize\" = 12.7"
equation "\"externalDiameter\" = 28.575"
equation "\"thickness\" = 9.525"
equation "\"printSpacing\" = 0.5715"
body "Solid1"
